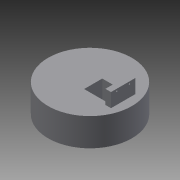
# Autodesk Inventor part: manipulator base
Saved by Autodesk Inventor 2015 (Build 190159000, 159)
## iProperties
Created: 2014-10-18
Part Number: manipulator base
Material: Generic
Document SubType Name: Modeling
Designer: ericd_000
Density: 1 g/cm^3
Appearance: Default
Author: ericd_000
Autodesk Inventor part; units mm, degrees
ref_plane "YZ Plane" through (0, 0, 0) normal (1, 0, 0) x (0, 1, 0)
ref_plane "XZ Plane" through (0, 0, 0) normal (0, 1, 0) x (-1, 0, 0)
ref_plane "XY Plane" through (0, 0, 0) normal (0, 0, 1) x (1, 0, 0)
sketch "Sketch1" plane through (0, 0, 0) normal (0, 0, 1) x (1, 0, 0)
  circle A0 centre (0, 0) radius 60
  dimension "d0" = 120
  constraints: 1 centre point, 1 coincident
  measures "d0" diameter of A0
extrude "Extrusion1" add sketch "Sketch1" along normal blind 40
sketch "Sketch4" plane through (0, 0, 40) normal (0, 0, 1) x (1, 0, 0)
  line L0 (4.6, 13) -> (39.6, 13)
  line L1 (39.6, 13) -> (39.6, -13)
  line L2 (39.6, -13) -> (4.6, -13)
  line L3 (4.6, -13) -> (4.6, 13)
  line L4 (0, 0) -> (4.6, 0) construction
  dimension "d14" = 35
  dimension "d15" = 26
  dimension "d16" = 4.6
  constraints: 10 end point, 2 horizontal, 2 parallel, 1 horizontal alignment, 1 midpoint, 1 perpendicular
  measures "d14" distance of L0.start L0.end
  measures "d15" distance of L0.end L1.end
  measures "d16" distance of L4.start L4.end
extrude "Extrusion4" cut sketch "Sketch4" against normal blind 30
sketch "Sketch5" plane through (0, 0, 40) normal (0, 0, 1) x (1, 0, 0)
  line L0 (47.6, -17.5) -> (39.6, -17.5)
  line L1 (39.6, -17.5) -> (39.6, 17.5)
  line L2 (39.6, 17.5) -> (47.6, 17.5)
  line L3 (47.6, 17.5) -> (47.6, -17.5)
  line L4 (39.6, 13) -> (39.6, -13) projected
  point P0 (0, 0)
  point P1 (39.6, 0)
  point P2 (39.6, 0)
  dimension "d19" = 35
  dimension "d20" = 8
  constraints: 8 end point, 2 midpoint, 2 parallel, 1 coincident, 1 horizontal, 1 horizontal alignment, 1 perpendicular
  measures "d19" distance of L2.end L0.start
  measures "d20" distance of L0.start L0.end
extrude "Extrusion5" add sketch "Sketch5" along normal blind 20
sketch "Sketch6" plane through (39.6, -13, 10) normal (-1, 0, 0) x (0, 0, 1)
  circle A0 centre (47, 22) radius 1
  circle A1 centre (47, 4) radius 1
  line L0 (47, 22) -> (47, 4) construction
  line L1 (50, 30.5) -> (50, -4.5) construction
  point P0 (-10, 13)
  point P1 (47, 13)
  point P2 (50, 13)
  dimension "d23" = 18
  dimension "d24" = 2
  dimension "d25" = 2
  dimension "d26" = 3
  constraints: 2 centre point, 2 end point, 2 midpoint, 1 horizontal alignment, 1 parallel
  measures "d23" distance of L0.start L0.end
  measures "d24" diameter of A0
  measures "d25" diameter of A1
  measures "d26" distance between parallel lines of L1 L0
extrude "Extrusion6" cut sketch "Sketch6" against normal up to surface (8 mm away)
body "Solid1"
